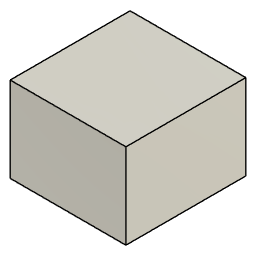
Printer-V1 (Autodesk Fusion 360 design; units mm, degrees)
Autodesk Fusion 360 part; units mm, degrees
sketch "Skizze1" plane through (0, 0, 0) normal (0, 0, 1) x (1, 0, 0)
  line L0 (-42.5691, 34.1396) -> (317.4309, 34.1396)
  line L1 (317.4309, 34.1396) -> (317.4309, -338.8604)
  line L2 (317.4309, -338.8604) -> (-42.5691, -338.8604)
  line L3 (-42.5691, -338.8604) -> (-42.5691, 34.1396)
  dimension "d1" = 360
  dimension "d2" = 373
  constraint horizontal L0
  constraint vertical L1
  constraint horizontal L2
  constraint vertical L3
  measures "d1" distance of L0.start L0.end
  measures "d2" distance of L0.start L2.end
extrude "Extrusion1" add sketch "Skizze1" along normal blind 265
named bodies: "printer"
